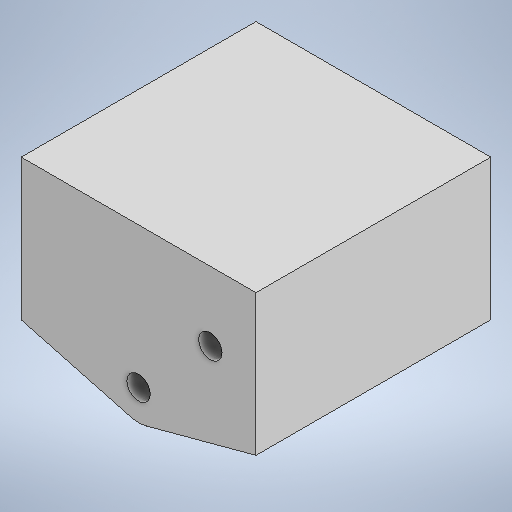
# Autodesk Inventor part: Корпус
Saved by Autodesk Inventor 2025 (Build 290162010, 162A)
## iProperties
Created: 2024-06-14
Part Number: Корпус
Material: Типовые
Document SubType Name: Modeling
Designer: Edward_Higgins
Density: 1 g/cm^3
Appearance: По умолчанию
Author: Edward_Higgins
Autodesk Inventor part; units mm, degrees
ref_plane "YZ Plane" through (0, 0, 0) normal (1, 0, 0) x (0, 1, 0)
ref_plane "XZ Plane" through (0, 0, 0) normal (0, 1, 0) x (-1, 0, 0)
ref_plane "XY Plane" through (0, 0, 0) normal (0, 0, 1) x (1, 0, 0)
sketch "Эскиз1" plane through (0, 0, 0) normal (0, 0, 1) x (1, 0, 0)
  line L0 (-125, 150) -> (125, 150)
  line L1 (125, 150) -> (125, 0)
  line L2 (125, 0) -> (-125, 0) construction
  line L3 (-125, 0) -> (-125, 150)
  circle A0 centre (0, 0) radius 12.5
  circle A1 centre (76.3675, 76.3675) radius 12.5
  line L4 (0, 0) -> (76.3675, 76.3675) construction
  line L5 (-125, 0) -> (-8.3734, -31.25)
  arc A2 (-8.3734, -31.25) -> (8.3734, -31.25) centre (0, 0) ccw
  line L6 (8.3734, -31.25) -> (125, 0)
  dimension "d0" = 108
  dimension "d3" = 45
  dimension "d4" = 250
  dimension "d5" = 150
  dimension "d6" = 25
  dimension "d7" = 15
  constraints: 14 end point, 3 centre point, 3 coincident, 2 parallel, 2 point on circle, 2 tangent, 1 equal radius, 1 horizontal, 1 midpoint, 1 perpendicular
  measures "d0" distance of L4.start L4.end
  measures "d3" angle of L2 L4
  measures "d4" distance between parallel lines of L1 L3
  measures "d5" distance from line of point (0, 0) L0
  measures "d6" diameter of A0
  measures "d7" angle of L2 L5
extrude "Выдавливание1" add sketch "Эскиз1" along normal mid plane 250
